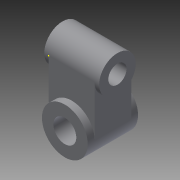
# Autodesk Inventor part: HW 6 Part 5
Saved by Autodesk Inventor 2015 (Build 190159000, 159)
## iProperties
Created: 2016-02-15
Part Number: HW 6 Part 5
Material: Generic
Document SubType Name: Modeling
Designer: Melissa
Density: 1 g/cm^3
Appearance: Default
Author: Melissa
Autodesk Inventor part; units mm, degrees
ref_plane "YZ Plane" through (0, 0, 0) normal (1, 0, 0) x (0, 1, 0)
ref_plane "XZ Plane" through (0, 0, 0) normal (0, 1, 0) x (-1, 0, 0)
ref_plane "XY Plane" through (0, 0, 0) normal (0, 0, 1) x (1, 0, 0)
sketch "Sketch1" plane through (0, 0, 0) normal (0, 0, 1) x (1, 0, 0)
  line L0 (0, 0) -> (63.5, 0)
  line L1 (63.5, 0) -> (63.5, -69.85)
  line L2 (63.5, -69.85) -> (0, -69.85)
  line L3 (0, -69.85) -> (0, 0)
  dimension "d0" = 63.5
  dimension "d1" = 69.85
  dimension "d2" = 63.5
  constraints: 8 end point, 2 perpendicular, 1 horizontal
  measures "d0" distance of L0.start L0.end
  measures "d1" distance of L0.end L1.end
  measures "d2" distance of L1.end L2.end
extrude "Extrusion1" add sketch "Sketch1" along normal blind 50.8
sketch "Sketch2" plane through (0, 0, 50.8) normal (0, 0, 1) x (1, 0, 0)
  line L0 (0, -69.85) -> (63.5, -69.85) projected
  circle A0 centre (31.75, -69.85) radius 31.75
  circle A1 centre (31.75, -69.85) radius 15.875
  point P0 (0, 0)
  dimension "d5" = 31.75
  constraints: 1 centre point, 1 coincident, 1 horizontal alignment, 1 midpoint, 2 other
  measures "d5" diameter of A1
extrude "Extrusion2" add sketch "Sketch2" along normal blind 9.525 and the other way blind 60.325 contours A1 L0 A0 | L0 A0 A1
sketch "Sketch3" plane through (63.5, 0, 50.8) normal (1, 0, 0) x (0, 0, -1)
  point P0 (50.8, 0)
sketch "Sketch4" plane through (0, 0, 50.8) normal (0, 0, 1) x (1, 0, 0)
  line L0 (47.625, -69.85) -> (15.875, -69.85) projected
  circle A0 centre (31.75, -69.85) radius 15.875
  point P0 (0, 0)
  dimension "d10" = 31.75
  constraints: 1 centre point, 1 midpoint
  measures "d10" diameter of A0
sketch "Sketch5" plane through (0, 0, 50.8) normal (0, 0, 1) x (1, 0, 0)
  point P0 (0, 0)
extrude "Extrusion3" cut sketch "Sketch4" against normal through all
sketch "Sketch6" plane through (63.5, 0, 50.8) normal (1, 0, 0) x (0, 0, -1)
  line L0 (50.8, 0) -> (0, 0) projected
  circle A0 centre (25.4, 0) radius 25.4
  dimension "d13" = 50.8
  constraints: 1 centre point, 1 midpoint
  measures "d13" diameter of A0
extrude "Extrusion4" add sketch "Sketch6" along normal blind 6.35 and the other way blind 69.85
sketch "Sketch7" plane through (69.85, 0, 25.4) normal (1, 0, 0) x (0, 0, -1)
  circle A0 centre (0, 0) radius 12.7
  point P0 (25.4, 0)
  dimension "d18" = 25.4
  constraints: 1 centre point
  measures "d18" diameter of A0
extrude "Extrusion5" cut sketch "Sketch7" against normal through all
body "Solid1"
